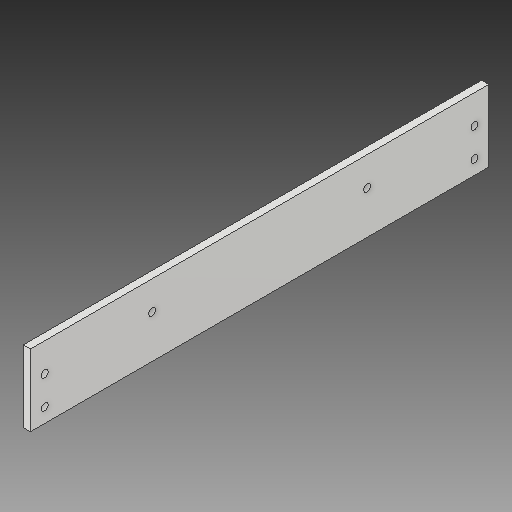
# Autodesk Inventor part: 15102898-16-P-0403
Saved by Autodesk Inventor 2017 (Build 210142000, 142)
## iProperties
Created: 2016-10-08
Part Number: 15102898-16-P-0403
Material: LCP Plastic
Document SubType Name: Modeling
Designer: gus
Density: 1.626 g/cm^3
Appearance: Smooth - White
Mass: 264.492 g
Surface Area: 579.606 cm^2
Volume: 162.664 cm^3
Author: gus
Autodesk Inventor part; units mm, degrees
ref_plane "YZ Plane" through (0, 0, 0) normal (1, 0, 0) x (0, 1, 0)
ref_plane "XZ Plane" through (0, 0, 0) normal (0, 1, 0) x (-1, 0, 0)
ref_plane "XY Plane" through (0, 0, 0) normal (0, 0, 1) x (1, 0, 0)
sketch "Sketch1" plane through (0, 0, 0) normal (1, 0, 0) x (0, 1, 0)
  line L0 (0, 0) -> (63.5, 0)
  line L1 (63.5, 0) -> (63.5, 406.4)
  line L2 (63.5, 406.4) -> (0, 406.4)
  line L3 (0, 406.4) -> (0, 0)
  circle A0 centre (38.1, 393.7) radius 3.175
  circle A1 centre (12.7, 393.7) radius 3.175
  circle A2 centre (38.1, 12.7) radius 3.175
  circle A3 centre (12.7, 12.7) radius 3.175
  dimension "d0" = 63.5
  dimension "d1" = 406.4
  dimension "d2" = 6.35
  dimension "d3" = 6.35
  dimension "d4" = 6.35
  dimension "d5" = 6.35
  dimension "d6" = 12.7
  dimension "d7" = 12.7
  dimension "d8" = 12.7
  dimension "d9" = 25.4
  dimension "d10" = 25.4
  dimension "d11" = 12.7
  dimension "d12" = 12.7
  dimension "d13" = 25.4
  constraints: 8 end point, 4 centre point, 2 parallel, 1 horizontal, 1 perpendicular
  measures "d0" distance of L2.end L1.end
  measures "d1" distance of L1.end L0.end
  measures "d2" diameter of A0
  measures "d3" diameter of A1
  measures "d4" diameter of A2
  measures "d5" diameter of A3
  measures "d6" distance from line of L2 A0.centre
  measures "d7" distance from line of L2 A1.centre
  measures "d8" distance from line of L3 A1.centre
  measures "d9" distance from line of L1 A0.centre
  measures "d10" distance of A3.centre A2.centre
  measures "d11" distance from line of L0 A2.centre
  measures "d12" distance from line of L0 A3.centre
  measures "d13" distance from line of L1 A2.centre
extrude "Extrusion1" add sketch "Sketch1" along normal blind 6.35
sketch "Sketch2" plane through (0, 0, 0) normal (-1, 0, 0) x (0, 0, 1)
  circle A0 centre (107.95, 38.1) radius 3.175
  circle A1 centre (298.45, 38.1) radius 3.175
  line L0 (0, 63.5) -> (406.4, 63.5) projected
  line L1 (0, 0) -> (0, 63.5) projected
  line L2 (406.4, 63.5) -> (406.4, 0) projected
  dimension "d16" = 6.35
  dimension "d17" = 6.35
  dimension "d18" = 25.4
  dimension "d19" = 25.4
  dimension "d20" = 107.95
  dimension "d21" = 107.95
  constraints: 2 centre point
  measures "d16" diameter of A0
  measures "d17" diameter of A1
  measures "d18" distance from line of L0 A0.centre
  measures "d19" distance from line of L0 A1.centre
  measures "d20" distance from line of L1 A0.centre
  measures "d21" distance from line of L2 A1.centre
extrude "Extrusion2" cut sketch "Sketch2" against normal blind 6.35
body "Solid1"
